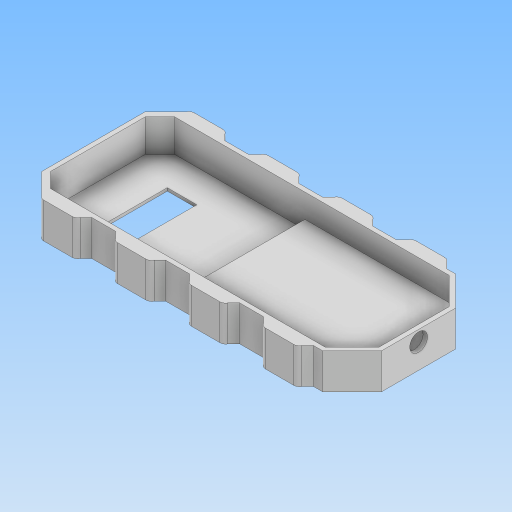
# Autodesk Inventor part: RC5 Controller
Saved by Autodesk Inventor 2024 (Build 280153000, 153)
## iProperties
Created: 2024-03-14
Part Number: RC5 Controller
Material: Generic
Document SubType Name: Modeling
Designer: MenMe
Density: 1 g/cm^3
Appearance: Default
Author: MenMe
Autodesk Inventor part; units mm, degrees
ref_plane "YZ Plane" through (0, 0, 0) normal (1, 0, 0) x (0, 1, 0)
ref_plane "XZ Plane" through (0, 0, 0) normal (0, 1, 0) x (-1, 0, 0)
ref_plane "XY Plane" through (0, 0, 0) normal (0, 0, 1) x (1, 0, 0)
sketch "Sketch1" plane through (0, 0, 0) normal (0, 1, 0) x (-1, 0, 0)
  line L0 (110, 0) -> (110, -45)
  line L1 (110, -45) -> (10, -45)
  line L2 (10, -45) -> (0, -35)
  line L3 (0, -35) -> (0, -10)
  line L4 (0, -10) -> (10, 0)
  line L5 (110, 0) -> (10, 0)
  line L6 (28, 0) -> (28, 3)
  line L7 (28, 3) -> (15, 3)
  line L8 (15, 3) -> (15, 0)
  line L9 (53, 0) -> (53, 3)
  line L10 (53, 3) -> (40, 3)
  line L11 (40, 3) -> (40, 0)
  line L12 (78, 0) -> (78, 3)
  line L13 (78, 3) -> (65, 3)
  line L14 (65, 3) -> (65, 0)
  line L15 (103, 0) -> (103, 3)
  line L16 (103, 3) -> (90, 3)
  line L17 (90, 3) -> (90, 0)
  line L18 (28, -45) -> (28, -48)
  line L19 (28, -48) -> (15, -48)
  line L20 (15, -48) -> (15, -45)
  line L21 (53, -45) -> (53, -48)
  line L22 (53, -48) -> (40, -48)
  line L23 (40, -48) -> (40, -45)
  line L24 (78, -45) -> (78, -48)
  line L25 (78, -48) -> (65, -48)
  line L26 (65, -48) -> (65, -45)
  line L27 (103, -45) -> (103, -48)
  line L28 (103, -48) -> (90, -48)
  line L29 (90, -48) -> (90, -45)
  point P0 (0, 0)
  point P1 (21.5, -48)
  point P2 (46.5, -48)
  point P3 (71.5, -48)
  point P4 (96.5, -48)
  point P5 (40, 0)
  point P6 (40, -45)
  point P7 (103, -45)
  point P8 (103, 0)
  point P9 (90, 0)
  point P10 (78, 0)
  point P11 (65, 0)
  point P12 (53, 0)
  dimension "d0" = 45
  dimension "d1" = 100
  dimension "d4" = 45
  dimension "d5" = 45
  dimension "d6" = 25
  dimension "d16" = 25
  dimension "d24" = 5
  dimension "d25" = 13
  dimension "d26" = 3
  dimension "d32" = 25
  dimension "d34" = 3
  dimension "d83" = 5
  constraints: 60 end point, 7 perpendicular, 6 point on line, 3 equal length, 2 horizontal, 1 midpoint, 1 parallel, 46 other
  measures "d0" distance of L0.start L0.end
  measures "d1" distance of L0.end L1.end
  measures "d4" angle of L2 L3
  measures "d5" angle of L4 L3
  measures "d6" distance of L2.end L3.end
  measures "d16" distance of L6.start L9.start
  measures "d24" distance from line of L1.end L20
  measures "d25" distance of L18.end L19.end
  measures "d26" distance from line of L1 point (21.5, -48)
  measures "d32" distance of L18.start L21.start
  measures "d34" distance between parallel lines of L5 L7
  measures "d83" distance from line of L4.end L8
extrude "Extrusion1" add sketch "Sketch1" along normal blind 12
sketch "Sketch2" plane through (0, 12, 0) normal (0, 1, 0) x (1, 0, 0)
  line L0 (-40, -3) -> (-40, 0) projected
  line L1 (-40, 0) -> (-28, 0) projected
  line L2 (-28, 0) -> (-28, -3) projected
  line L3 (-28, -3) -> (-15, -3) projected
  line L4 (-15, -3) -> (-15, 0) projected
  line L5 (-15, 0) -> (-10, 0) projected
  line L6 (-10, 0) -> (0, 10) projected
  line L7 (0, 10) -> (0, 35) projected
  line L8 (0, 35) -> (-10, 45) projected
  line L9 (-10, 45) -> (-15, 45) projected
  line L10 (-15, 45) -> (-15, 48) projected
  line L11 (-15, 48) -> (-28, 48) projected
  line L12 (-28, 48) -> (-28, 45) projected
  line L13 (-28, 45) -> (-40, 45) projected
  line L14 (-40, 45) -> (-40, 48) projected
  line L15 (-40, 48) -> (-53, 48) projected
  line L16 (-53, 48) -> (-53, 45) projected
  line L17 (-53, 45) -> (-65, 45) projected
  line L18 (-65, 45) -> (-65, 48) projected
  line L19 (-65, 48) -> (-78, 48) projected
  line L20 (-78, 48) -> (-78, 45) projected
  line L21 (-78, 45) -> (-90, 45) projected
  line L22 (-90, 45) -> (-90, 48) projected
  line L23 (-90, 48) -> (-103, 48) projected
  line L24 (-103, 48) -> (-103, 45) projected
  line L25 (-103, 45) -> (-110, 45) projected
  line L26 (-110, 45) -> (-110, 0) projected
  line L27 (-110, 0) -> (-103, 0) projected
  line L28 (-103, 0) -> (-103, -3) projected
  line L29 (-103, -3) -> (-90, -3) projected
  line L30 (-90, -3) -> (-90, 0) projected
  line L31 (-90, 0) -> (-78, 0) projected
  line L32 (-78, 0) -> (-78, -3) projected
  line L33 (-78, -3) -> (-65, -3) projected
  line L34 (-65, -3) -> (-65, 0) projected
  line L35 (-65, 0) -> (-53, 0) projected
  line L36 (-53, 0) -> (-53, -3) projected
  line L37 (-53, -3) -> (-40, -3) projected
  line L38 (-1.5, 34.3787) -> (-1.5, 10.6213)
  line L39 (-1.5, 10.6213) -> (-10.6213, 1.5)
  line L40 (-10.6213, 1.5) -> (-21, 1.5)
  line L41 (-21, 1.5) -> (-46, 1.5)
  line L42 (-46, 1.5) -> (-71, 1.5)
  line L43 (-71, 1.5) -> (-96, 1.5)
  line L44 (-96, 1.5) -> (-108.5, 1.5)
  line L45 (-108.5, 1.5) -> (-108.5, 43.5)
  line L46 (-108.5, 43.5) -> (-97, 43.5)
  line L47 (-97, 43.5) -> (-72, 43.5)
  line L48 (-72, 43.5) -> (-47, 43.5)
  line L49 (-47, 43.5) -> (-22, 43.5)
  line L50 (-22, 43.5) -> (-10.6213, 43.5)
  line L51 (-10.6213, 43.5) -> (-1.5, 34.3787)
  line L52 (-110.2223, -59.5852) -> (-109.4363, 98.5998) construction
  line L53 (-109.4363, 98.5998) -> (22.9503, 97.942) construction
  line L54 (22.9503, 97.942) -> (22.1643, -60.243) construction
  line L55 (22.1643, -60.243) -> (-110.2223, -59.5852) construction
  point P0 (0, 0)
  dimension "d58" = 42
  constraints: 28 end point, 15 other
  measures "d58" distance of L44.end L45.end
extrude "Extrusion2" cut sketch "Sketch2" against normal blind 11 contours L38 L39 L40 L41 L42 L43 L44 L45 L46 L47 L48 L49 L50 L51
chamfer "Chamfer1" distance 2 angle 45 16 edges at (-53, 6, 0) (-40, 6, 0) (-65, 6, 0) (-78, 6, 0) (-90, 6, 0) (-103, 6, 0) (-28, 6, 0) (-15, 6, 0) (-15, 6, -45) (-28, 6, -45) (-40, 6, -45) (-53, 6, -45) (-65, 6, -45) (-78, 6, -45) (-90, 6, -45) (-103, 6, -45)
chamfer "Chamfer2" distance 5 angle 45 4 edges at (-110, 6, -45) (-110, 6, 0) (-108.5, 6.5, -43.5) (-108.5, 6.5, -1.5)
sketch "Sketch3" plane through (0, 0, -10) normal (1, 0, 0) x (0, 0, -1)
  line L0 (0, 0) -> (0, 12) projected
  line L1 (25, 0) -> (25, 12) projected
  line L2 (0, 0) -> (25, 0) projected
  circle A0 centre (12.5, 8.3) radius 3
  point P0 (-10, 0)
  dimension "d93" = 6
  dimension "d94" = 12.5
  dimension "d95" = 8.3
  constraints: 1 centre point
  measures "d93" diameter of A0
  measures "d94" distance from line of L1 A0.centre
  measures "d95" distance from line of L2 A0.centre
extrude "Extrusion3" cut sketch "Sketch3" against normal blind 8
fillet "Fillet1" radius 2 16 edges at (-53, 6, -48) (-40, 6, -48) (-28, 6, -48) (-15, 6, -48) (-65, 6, -48) (-78, 6, -48) (-90, 6, -48) (-103, 6, -48) (-15, 6, 3) (-28, 6, 3) (-40, 6, 3) (-53, 6, 3) (-65, 6, 3) (-78, 6, 3) (-90, 6, 3) (-103, 6, 3)
sketch "Sketch5" plane through (0, 1, 0) normal (0, 1, 0) x (1, 0, 0)
  line L0 (-103.5, 43.5) -> (-10.6213, 43.5) projected
  line L1 (-10.6213, 1.5) -> (-103.5, 1.5) projected
  line L2 (-108.5, 6.5) -> (-103.5, 1.5) projected
  line L3 (-10.6213, 1.5) -> (-103.5, 1.5) projected
  line L4 (-1.5, 10.6213) -> (-10.6213, 1.5) projected
  line L5 (-1.5, 34.3787) -> (-1.5, 10.6213) projected
  line L6 (-10.6213, 43.5) -> (-1.5, 34.3787) projected
  line L7 (-103.5, 43.5) -> (-10.6213, 43.5) projected
  line L8 (-103.5, 43.5) -> (-108.5, 38.5) projected
  line L9 (-108.5, 6.5) -> (-108.5, 38.5) projected
  line L10 (-10.6213, 1.5) -> (-1.5, 10.6213)
  line L11 (-1.5, 34.3787) -> (-1.5, 10.6213)
  line L12 (-1.5, 34.3787) -> (-10.6213, 43.5)
  line L13 (-10.6213, 43.5) -> (-59.4466, 43.5)
  line L14 (-59.4466, 43.5) -> (-59.4466, 1.5)
  line L15 (-59.4466, 1.5) -> (-10.6213, 1.5)
  point P0 (0, 0)
  point P1 (-59.4466, 1.5)
  point P2 (-10.6213, 43.5)
  constraints: 12 end point, 3 perpendicular, 2 collinear, 2 point on line
extrude "Extrusion4" add sketch "Sketch5" along normal blind 3 contours L0 L6 L5 L4 L1 L14
sketch "Sketch6" plane through (0, 0, 0) normal (0, -1, 0) x (1, 0, 0)
  line L0 (-95, -32.5) -> (-85, -32.5)
  line L1 (-85, -32.5) -> (-85, -12.5)
  line L2 (-85, -12.5) -> (-95, -12.5)
  line L3 (-95, -12.5) -> (-95, -32.5)
  line L4 (-110, -40) -> (-110, -5) projected
  line L5 (-80, -45) -> (-88, -45) projected
  point P0 (0, 0)
  point P1 (-110, -22.5)
  point P2 (-84, -45)
  dimension "d102" = 10
  dimension "d103" = 20
  dimension "d104" = 15
  dimension "d106" = 12.5
  constraints: 8 end point, 2 midpoint, 2 parallel, 1 horizontal, 1 perpendicular
  measures "d102" distance of L1.end L2.end
  measures "d103" distance of L2.end L0.start
  measures "d104" distance from line of point (-110, -22.5) L3
  measures "d106" distance from line of point (-84, -45) L0
extrude "Extrusion5" cut sketch "Sketch6" against normal blind 3
body "Solid1"
